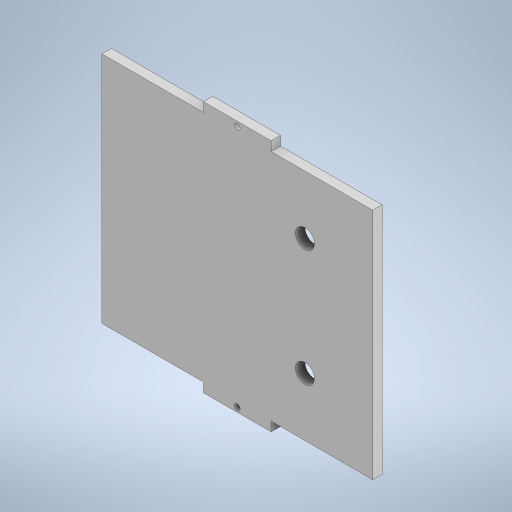
# Autodesk Inventor part: broomba base
Saved by Autodesk Inventor 2023.2 (Build 272271000, 271)
## iProperties
Created: 2023-07-21
Part Number: broomba base
Material: Generic
Document SubType Name: Modeling
Designer: 30067459
Density: 1 g/cm^3
Appearance: Default
Author: 30067459
Autodesk Inventor part; units mm, degrees
ref_plane "YZ Plane" through (0, 0, 0) normal (1, 0, 0) x (0, 1, 0)
ref_plane "XZ Plane" through (0, 0, 0) normal (0, 1, 0) x (-1, 0, 0)
ref_plane "XY Plane" through (0, 0, 0) normal (0, 0, 1) x (1, 0, 0)
sketch "Sketch1" plane through (0, 0, 0) normal (0, 0, 1) x (1, 0, 0)
  line L0 (72.5, 62.5) -> (-72.5, 62.5)
  line L1 (-72.5, 62.5) -> (-72.5, -62.5)
  line L2 (-72.5, -62.5) -> (72.5, -62.5)
  line L3 (72.5, -62.5) -> (72.5, 62.5)
  line L4 (72.5, 62.5) -> (-72.5, -62.5) construction
  line L5 (-72.5, 62.5) -> (72.5, -62.5) construction
  point P0 (0, 0)
  dimension "d0" = 145
  dimension "d1" = 125
  constraints: 12 end point, 2 midpoint, 2 parallel, 1 horizontal, 1 perpendicular
  measures "d0" distance of L2.end L1.end
  measures "d1" distance of L1.end L0.end
extrude "Extrusion1" add sketch "Sketch1" along normal blind 5
sketch "Sketch2" plane through (0, 0, 0) normal (0, 0, -1) x (-1, 0, 0)
  line L0 (-72.5, -62.5) -> (-72.5, 62.5) projected
  line L1 (-72.5, 62.5) -> (0, 0)
  line L2 (0, 0) -> (-72.5, -62.5)
  circle A0 centre (-36.25, 31.25) radius 5
  circle A1 centre (-36.25, -31.25) radius 5
  dimension "d4" = 10
  dimension "d5" = 10
  constraints: 4 end point, 2 centre point, 2 midpoint
  measures "d4" diameter of A0
  measures "d5" diameter of A1
extrude "Extrusion2" cut sketch "Sketch2" against normal blind 18.5 contours A1 L2 | L2 A1 | A0 L1 | L1 A0
sketch "Sketch3" plane through (0, 0, 0) normal (0, 0, -1) x (-1, 0, 0)
  line L0 (23.0298, -12.8396) -> (38.1112, -12.8396)
  line L1 (38.1112, -12.8396) -> (38.1112, 12.8396)
  line L2 (38.1112, 12.8396) -> (23.0298, 12.8396)
  line L3 (23.0298, 12.8396) -> (23.0298, -12.8396)
  line L4 (23.0298, -12.8396) -> (38.1112, 12.8396) construction
  line L5 (38.1112, -12.8396) -> (23.0298, 12.8396) construction
  point P0 (0, 0)
  point P1 (30.5705, 0)
  constraints: 12 end point, 2 midpoint, 2 parallel, 1 horizontal, 1 perpendicular
extrude "Extrusion3" add sketch "Sketch3" along normal blind 15
shell "Shell1" thickness 2 removed faces 1 at (-23.0298, 4.2799, -5)
sketch "Sketch4" plane through (0, 0, 5) normal (0, 0, 1) x (1, 0, 0)
  line L0 (-72.5, -62.5) -> (72.5, -62.5) projected
  line L1 (0, 0) -> (-72.5, -62.5)
  line L2 (-36.25, -31.25) -> (0, -62.5)
  line L3 (-36.25, -31.25) -> (-36.25, -62.5)
  line L4 (-18.125, -46.875) -> (-18.125, -62.5)
  line L5 (0, 0) -> (72.5, -62.5)
  circle A0 centre (36.25, -31.25) radius 5 projected
  line L6 (36.25, -31.25) -> (0, -62.5)
  line L7 (18.125, -46.875) -> (18.125, -62.5)
  line L8 (-18.125, -62.5) -> (18.125, -62.5)
  line L9 (18.125, -62.5) -> (18.125, -67.5)
  line L10 (18.125, -67.5) -> (-18.125, -67.5)
  line L11 (-18.125, -67.5) -> (-18.125, -62.5)
  dimension "d11" = 5
  constraints: 22 end point, 4 midpoint, 4 perpendicular, 3 point on line, 2 parallel, 1 horizontal
  measures "d11" distance of L8.end L9.end
extrude "Extrusion4" add sketch "Sketch4" against normal blind 5 contours L0 L9 L10 L11
sketch "Sketch5" plane through (0, 0, 5) normal (0, 0, 1) x (1, 0, 0)
  line L0 (72.5, -62.5) -> (72.5, 62.5) projected
  line L1 (0, 0) -> (72.5, 62.5)
  line L2 (-72.5, 62.5) -> (-72.5, -62.5) projected
  line L3 (0, 0) -> (-72.5, 62.5)
  circle A0 centre (36.25, 31.25) radius 5 projected
  line L4 (36.25, 31.25) -> (36.25, 62.5)
  line L5 (72.5, 62.5) -> (-72.5, 62.5) projected
  line L6 (-36.25, 31.25) -> (-36.25, 62.5)
  line L7 (-18.125, 15.625) -> (-18.125, 62.5)
  line L8 (36.25, 31.25) -> (0, 31.25)
  line L9 (18.125, 31.25) -> (18.125, 62.5)
  line L10 (18.125, 62.5) -> (-18.125, 62.5)
  line L11 (-18.125, 62.5) -> (-18.125, 67.5)
  line L12 (-18.125, 67.5) -> (18.125, 67.5)
  line L13 (18.125, 67.5) -> (18.125, 62.5)
  dimension "d14" = 5
  constraints: 22 end point, 4 point on line, 4 vertical, 2 horizontal, 2 midpoint, 2 parallel, 1 perpendicular
  measures "d14" distance of L10.end L11.end
extrude "Extrusion5" add sketch "Sketch5" against normal blind 5 contours L11 L12 L13 L5
sketch "Sketch6" plane through (0, 0, 5) normal (0, 0, 1) x (1, 0, 0)
  line L0 (-18.125, -62.5) -> (-18.125, -67.5) projected
  line L1 (18.125, -67.5) -> (18.125, -62.5) projected
  line L2 (-18.125, -62.5) -> (18.125, -62.5)
  circle A0 centre (0, -65) radius 1.5
  point P0 (0, 0)
  dimension "d17" = 3
  constraints: 2 end point, 1 centre point, 1 perpendicular
  measures "d17" diameter of A0
extrude "Extrusion6" cut sketch "Sketch6" against normal blind 2.75
sketch "Sketch7" plane through (0, 0, 5) normal (0, 0, 1) x (1, 0, 0)
  line L0 (-18.125, 62.5) -> (-72.5, 62.5) projected
  line L1 (18.125, 62.5) -> (18.125, 67.5) projected
  line L2 (-18.125, 62.5) -> (18.125, 62.5)
  circle A0 centre (0, 65) radius 1.5
  point P0 (0, 0)
  dimension "d20" = 3
  constraints: 2 end point, 1 centre point, 1 horizontal
  measures "d20" diameter of A0
extrude "Extrusion7" cut sketch "Sketch7" against normal blind 2.75
body "Solid1"
